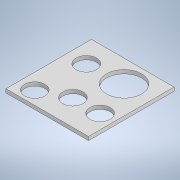
# Autodesk Inventor part: Bottle layout lower plate
Saved by Autodesk Inventor 2021 (Build 250183000, 183)
## iProperties
Created: 2020-07-28
Part Number: Bottle layout lower plate
Material: Generic
Document SubType Name: Modeling
Designer: jgray
Density: 1 g/cm^3
Appearance: Default
Author: jgray
Autodesk Inventor part; units mm, degrees
ref_plane "YZ Plane" through (0, 0, 0) normal (1, 0, 0) x (0, 1, 0)
ref_plane "XZ Plane" through (0, 0, 0) normal (0, 1, 0) x (-1, 0, 0)
ref_plane "XY Plane" through (0, 0, 0) normal (0, 0, 1) x (1, 0, 0)
sketch "Sketch1" plane through (0, 0, 0) normal (0, 1, 0) x (-1, 0, 0)
  line L0 (-56.25, 58.25) -> (56.25, 58.25)
  line L1 (56.25, 58.25) -> (56.25, -58.25)
  line L2 (56.25, -58.25) -> (-56.25, -58.25)
  line L3 (-56.25, -58.25) -> (-56.25, 58.25)
  line L4 (-56.25, 58.25) -> (56.25, -58.25) construction
  line L5 (56.25, 58.25) -> (-56.25, -58.25) construction
  point P0 (0, 0)
  dimension "d0" = 112.5
  dimension "d1" = 116.5
  constraints: 12 end point, 2 midpoint, 2 parallel, 1 horizontal, 1 perpendicular
  measures "d0" distance of L1.end L2.end
  measures "d1" distance of L0.end L1.end
extrude "Extrusion1" add sketch "Sketch1" along normal blind 5
sketch "Sketch2" plane through (0, 5, 0) normal (0, 1, 0) x (1, 0, 0)
  circle A0 centre (18.5, 27.9796) radius 23.85
  circle A1 centre (37, -23.25) radius 13.85
  circle A2 centre (-35, -40.25) radius 13.85
  circle A3 centre (-30.9, 25.8198) radius 13.85
  circle A4 centre (0, -23.25) radius 13.85
  line L0 (56.25, 58.25) -> (-56.25, 58.25) projected
  line L1 (-56.25, -58.25) -> (56.25, -58.25) projected
  line L2 (0, -105.9299) -> (0, 123.2086) construction
  line L3 (-76.4777, -40.25) -> (-5.35, -40.25) construction
  line L4 (-123.5447, -23.25) -> (82.5572, -23.25) construction
  line L5 (56.25, -58.25) -> (56.25, 58.25) construction
  point P0 (0, 0)
  dimension "d4" = 47.7
  dimension "d5" = 27.7
  dimension "d6" = 27.7
  dimension "d7" = 27.7
  dimension "d8" = 27.7
  dimension "d9" = 116.5
  dimension "d10" = 112.5
  dimension "d13" = 37
  dimension "d14" = 18.5
  dimension "d15" = 30.9
  dimension "d18" = 18
  dimension "d19" = 35
  dimension "d20" = 35
  constraints: 6 end point, 5 centre point, 3 point on line, 1 horizontal, 1 perpendicular, 1 vertical
  measures "d4" diameter of A0
  measures "d5" diameter of A1
  measures "d6" diameter of A2
  measures "d7" diameter of A3
  measures "d8" diameter of A4
  measures "d9" distance between parallel lines of L0 L1
  measures "d10" distance of L1.start L1.end
  measures "d13" distance of A4.centre A1.centre
  measures "d14" distance from line of A0.centre L2
  measures "d15" distance from line of A3.centre L2
  measures "d18" distance between parallel lines of L1 L3
  measures "d19" distance between parallel lines of L1 L4
  measures "d20" horizontal distance of A2.centre A4.centre
extrude "Extrusion2" cut sketch "Sketch2" against normal blind 5
body "Solid1"
